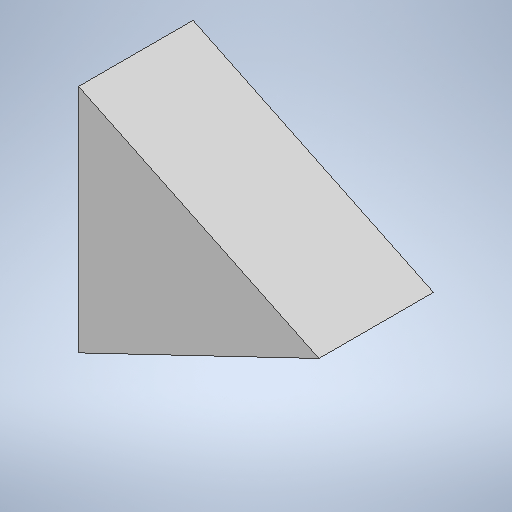
# Autodesk Inventor part: Triangle
Saved by Autodesk Inventor 2025.1 (Build 291241000, 241)
## iProperties
Created: 2025-04-04
Part Number: Triangle
Material: Generic
Document SubType Name: Modeling
Designer: victo
Density: 1 g/cm^3
Appearance: Default
Author: victo
Autodesk Inventor part; units mm, degrees
ref_plane "YZ Plane" through (0, 0, 0) normal (1, 0, 0) x (0, 1, 0)
ref_plane "XZ Plane" through (0, 0, 0) normal (0, 1, 0) x (-1, 0, 0)
ref_plane "XY Plane" through (0, 0, 0) normal (0, 0, 1) x (1, 0, 0)
sketch "Sketch1" plane through (0, 0, 0) normal (0, 0, 1) x (1, 0, 0)
  line L0 (0, 0) -> (-21, 10.0755)
  line L1 (-21, 10.0755) -> (-21, -10.0755)
  line L2 (-21, -10.0755) -> (0, 0)
  dimension "d0" = 21
  dimension "d1" = 10.0755
  dimension "d2" = 10.0755
  constraints: 6 end point, 1 vertical
  measures "d0" distance from line of L1 L0.start
  measures "d1" vertical distance of L0.start L1.end
  measures "d2" vertical distance of L0.end L0.start
extrude "Extrusion1" add sketch "Sketch1" along normal blind 10
equation "\"d2\" = d1"
body "Solid1"
